Autodesk Fusion 360 part; units mm, degrees
(part 7 of 18)
  line L4400 (196.1354, -58.294) -> (195.8306, -58.294)
  line L4401 (195.8306, -58.8002) -> (196.1354, -58.8002)
  line L4402 (195.8306, -56.7954) -> (196.1354, -56.7954)
  line L4403 (196.1354, -56.7954) -> (196.1354, -57.3016)
  line L4404 (195.8306, -57.3016) -> (195.8306, -56.7954)
  line L4405 (196.1354, -57.3016) -> (195.8306, -57.3016)
  line L4406 (198.9116, -20.2852) -> (198.9116, -20.6114)
  line L4407 (198.9116, -18.7589) -> (198.9116, -19.0849)
  line L4408 (196.0592, -18.7589) -> (198.9116, -18.7589)
  line L4409 (196.0592, -20.6114) -> (198.9116, -20.6114)
  line L4410 (196.514, -20.6112) -> (196.514, -18.7588)
  line L4411 (196.1354, -20.6874) -> (196.1354, -20.1812)
  line L4412 (196.1354, -20.1812) -> (195.8306, -20.1812)
  line L4413 (195.8306, -20.1812) -> (195.8306, -20.6874)
  line L4414 (195.8306, -20.6874) -> (196.1354, -20.6874)
  line L4415 (195.8306, -19.1888) -> (195.8306, -18.6826)
  line L4416 (195.8306, -18.6826) -> (196.1354, -18.6826)
  line L4417 (196.1354, -19.1888) -> (195.8306, -19.1888)
  line L4418 (196.1354, -18.6826) -> (196.1354, -19.1888)
  line L4419 (202.7186, -3.1004) -> (203.5186, -3.1004)
  line L4420 (202.1581, -3.1) -> (201.3582, -3.1)
  line L4421 (202.7186, -4.5201) -> (203.5186, -4.5201)
  line L4422 (202.1581, -4.5196) -> (201.3582, -4.5196)
  line L4423 (203.8283, -3.4103) -> (203.8283, -4.2103)
  line L4424 (201.0484, -4.2098) -> (201.0484, -3.4098)
  arc A623 (201.3582, -4.5196) -> (201.0484, -4.2098) centre (201.3583, -4.2097) cw
  arc A624 (201.0484, -3.4098) -> (201.3582, -3.1) centre (201.3583, -3.4099) cw
  arc A625 (203.5185, -3.1004) -> (203.8283, -3.4103) centre (203.5184, -3.4104) cw
  arc A626 (203.8283, -4.2102) -> (203.5185, -4.5201) centre (203.5184, -4.2102) cw
  line L4425 (200.8136, -6.0214) -> (201.6136, -6.0214)
  line L4426 (200.2531, -6.021) -> (199.4532, -6.021)
  line L4427 (200.8136, -7.4411) -> (201.6136, -7.4411)
  line L4428 (200.2531, -7.4406) -> (199.4532, -7.4406)
  line L4429 (201.9233, -6.3313) -> (201.9233, -7.1313)
  line L4430 (199.1434, -7.1308) -> (199.1434, -6.3308)
  arc A627 (199.4532, -7.4406) -> (199.1434, -7.1308) centre (199.4533, -7.1307) cw
  arc A628 (199.1434, -6.3308) -> (199.4532, -6.021) centre (199.4533, -6.3309) cw
  arc A629 (201.6135, -6.0214) -> (201.9233, -6.3313) centre (201.6134, -6.3314) cw
  arc A630 (201.9233, -7.1312) -> (201.6135, -7.4411) centre (201.6134, -7.1312) cw
  line L4431 (205.4602, -5.5356) -> (204.6602, -5.5356)
  line L4432 (206.0207, -5.536) -> (206.8207, -5.536)
  line L4433 (205.4602, -4.1159) -> (204.6602, -4.1159)
  line L4434 (206.0207, -4.1164) -> (206.8207, -4.1164)
  line L4435 (204.3505, -5.2258) -> (204.3505, -4.4257)
  line L4436 (207.1304, -4.4262) -> (207.1304, -5.2263)
  arc A631 (206.8206, -4.1164) -> (207.1304, -4.4262) centre (206.8205, -4.4263) cw
  arc A632 (207.1304, -5.2262) -> (206.8206, -5.536) centre (206.8205, -5.2261) cw
  arc A633 (204.6603, -5.5356) -> (204.3505, -5.2258) centre (204.6604, -5.2257) cw
  arc A634 (204.3505, -4.4258) -> (204.6603, -4.1159) centre (204.6605, -4.4259) cw
  line L4437 (-3.8371, -11.3611) -> (-0.0088, -11.3611)
  line L4438 (-0.009, 0.4389) -> (-3.8371, 0.439)
  line L4439 (8.163, 0.4389) -> (8.163, -11.3611)
  line L4440 (-3.837, -11.3611) -> (-3.8371, -8.5269)
  line L4441 (1.1469, -8.2551) -> (1.1469, -2.6671)
  line L4442 (-3.8371, -11.3611) -> (-0.0088, -11.3611)
  line L4443 (4.3347, -11.3611) -> (8.163, -11.3611)
  line L4444 (8.163, 0.4389) -> (4.3348, 0.4389)
  line L4445 (0.1309, -0.6731) -> (0.1309, -1.4861)
  line L4446 (4.1949, -0.6731) -> (4.1949, -1.4861)
  line L4447 (4.3347, -11.3611) -> (8.163, -11.3611)
  line L4448 (0.1309, -9.5124) -> (0.1309, -10.2489)
  line L4449 (4.1949, -10.2489) -> (4.1949, -9.2711)
  line L4450 (-3.8371, -7.4753) -> (-3.8371, -3.4469)
  line L4451 (-3.8371, -2.3953) -> (-3.8371, 0.4389)
  arc A635 (1.1469, -3.6831) -> (1.1469, -7.2391) centre (2.1413, -5.4611) cw
  line L4452 (195.842, -3.345) -> (195.842, -5.545)
  line L4453 (195.8344, -5.588) -> (196.8504, -5.588)
  line L4454 (196.8504, -5.588) -> (196.8504, -3.302)
  line L4455 (196.8504, -3.302) -> (195.8344, -3.302)
  arc A636 (195.3213, -3.1737) -> (195.0724, -3.1725) centre (195.1968, -3.1737) ccw
  arc A637 (195.0724, -3.175) -> (195.3213, -3.1737) centre (195.1968, -3.1737) ccw
  line L4456 (177.1674, -3.048) -> (172.3373, -3.048)
  line L4457 (177.1674, -5.588) -> (177.1674, -3.048)
  line L4458 (177.1674, -5.588) -> (172.3373, -5.588)
  line L4459 (172.3373, -5.588) -> (172.3373, -3.048)
  line L4460 (181.2044, -1.3566) -> (181.2044, -3.0235)
  line L4461 (181.2044, 2.4608) -> (181.2044, 0.9765)
  line L4462 (190.1444, -1.3566) -> (190.1444, -3.0235)
  line L4463 (190.1444, 2.411) -> (190.1444, 0.9765)
  line L4464 (181.2044, 2.4608) -> (190.1444, 2.411)
  line L4465 (200.2342, -1.2444) -> (199.2753, -1.2444)
  line L4466 (199.2753, -1.2444) -> (199.2753, -2.5656)
  line L4467 (199.2753, -2.5656) -> (200.2342, -2.5656)
  line L4468 (201.0866, -1.2444) -> (202.0455, -1.2444)
  line L4469 (202.0455, -1.2444) -> (202.0455, -2.5656)
  line L4470 (202.0455, -2.5656) -> (201.0866, -2.5656)
  line L4471 (213.977, -5.1867) -> (214.6507, -5.1867)
  line L4472 (214.6507, -5.1867) -> (214.6507, -5.8604)
  line L4473 (213.977, -12.3392) -> (214.6507, -12.3392)
  line L4474 (214.6507, -12.3392) -> (214.6507, -11.6655)
  line L4475 (208.172, -5.1867) -> (207.4983, -5.1867)
  line L4476 (207.4983, -5.1867) -> (207.4983, -5.8604)
  line L4477 (208.172, -12.3392) -> (207.4983, -12.3392)
  line L4478 (207.4983, -12.3392) -> (207.4983, -11.6655)
  arc A638 (207.1096, -6.1629) -> (206.9597, -6.1629) centre (207.0347, -6.1629) ccw
  arc A639 (206.9597, -6.1629) -> (207.1096, -6.1629) centre (207.0347, -6.1629) ccw
  line L4479 (188.1326, -7.3916) -> (189.0915, -7.3916)
  line L4480 (189.0915, -7.3916) -> (189.0915, -6.0704)
  line L4481 (189.0915, -6.0704) -> (188.1326, -6.0704)
  line L4482 (187.2802, -7.3916) -> (186.3213, -7.3916)
  line L4483 (186.3213, -7.3916) -> (186.3213, -6.0704)
  line L4484 (186.3213, -6.0704) -> (187.2802, -6.0704)
  line L4485 (182.7082, -6.0704) -> (181.7493, -6.0704)
  line L4486 (181.7493, -6.0704) -> (181.7493, -7.3916)
  line L4487 (181.7493, -7.3916) -> (182.7082, -7.3916)
  line L4488 (183.5606, -6.0704) -> (184.5195, -6.0704)
  line L4489 (184.5195, -6.0704) -> (184.5195, -7.3916)
  line L4490 (184.5195, -7.3916) -> (183.5606, -7.3916)
  line L4491 (208.6489, -3.8645) -> (208.6489, -0.7644)
  line L4492 (211.749, -0.7644) -> (208.6489, -0.7644)
  line L4493 (211.7477, -3.8645) -> (211.7477, -0.7644)
  line L4494 (208.6489, -3.8886) -> (209.4871, -3.8886)
  line L4495 (210.9095, -3.8886) -> (211.7477, -3.8886)
  arc A640 (209.5125, -3.8886) -> (210.9095, -3.8886) centre (210.211, -4.1061) cw
  arc A641 (212.2667, -3.8099) -> (212.0665, -3.8099) centre (212.1666, -3.8099) ccw
  arc A642 (212.0665, -3.8099) -> (212.2667, -3.8099) centre (212.1666, -3.8099) ccw
  line L4496 (141.7615, -77.4607) -> (141.7615, -77.7869)
  line L4497 (141.7615, -75.9344) -> (141.7615, -76.2604)
  line L4498 (138.9091, -75.9344) -> (141.7615, -75.9344)
  line L4499 (138.9091, -77.7869) -> (141.7615, -77.7869)
  line L4500 (139.3639, -77.7867) -> (139.3639, -75.9343)
  line L4501 (138.9853, -77.863) -> (138.9853, -77.3568)
  line L4502 (138.6805, -77.3568) -> (138.6805, -77.863)
  line L4503 (138.9853, -77.3568) -> (138.6805, -77.3568)
  line L4504 (138.6805, -77.863) -> (138.9853, -77.863)
  line L4505 (138.6805, -76.3644) -> (138.6805, -75.8582)
  line L4506 (138.9853, -75.8582) -> (138.9853, -76.3644)
  line L4507 (138.6805, -75.8582) -> (138.9853, -75.8582)
  line L4508 (138.9853, -76.3644) -> (138.6805, -76.3644)
  line L4509 (141.7615, -20.2852) -> (141.7615, -20.6114)
  line L4510 (141.7615, -18.7589) -> (141.7615, -19.0849)
  line L4511 (138.9091, -18.7589) -> (141.7615, -18.7589)
  line L4512 (138.9091, -20.6114) -> (141.7615, -20.6114)
  line L4513 (139.3639, -20.6112) -> (139.3639, -18.7588)
  line L4514 (138.6805, -20.6874) -> (138.9853, -20.6874)
  line L4515 (138.9853, -20.1812) -> (138.6805, -20.1812)
  line L4516 (138.6805, -20.1812) -> (138.6805, -20.6874)
  line L4517 (138.9853, -20.6874) -> (138.9853, -20.1812)
  line L4518 (138.6805, -19.1888) -> (138.6805, -18.6826)
  line L4519 (138.9853, -18.6826) -> (138.9853, -19.1888)
  line L4520 (138.6805, -18.6826) -> (138.9853, -18.6826)
  line L4521 (138.9853, -19.1888) -> (138.6805, -19.1888)
  line L4522 (141.7615, -39.3352) -> (141.7615, -39.6614)
  line L4523 (141.7615, -37.8089) -> (141.7615, -38.135)
  line L4524 (138.9091, -37.8089) -> (141.7615, -37.8089)
  line L4525 (138.9091, -39.6614) -> (141.7615, -39.6614)
  line L4526 (139.3639, -39.6613) -> (139.3639, -37.8089)
  line L4527 (138.6805, -39.2313) -> (138.6805, -39.7375)
  line L4528 (138.9853, -39.7375) -> (138.9853, -39.2313)
  line L4529 (138.6805, -39.7375) -> (138.9853, -39.7375)
  line L4530 (138.9853, -39.2313) -> (138.6805, -39.2313)
  line L4531 (138.6805, -38.2389) -> (138.6805, -37.7327)
  line L4532 (138.9853, -38.2389) -> (138.6805, -38.2389)
  line L4533 (138.9853, -37.7327) -> (138.9853, -38.2389)
  line L4534 (138.6805, -37.7327) -> (138.9853, -37.7327)
  line L4535 (141.7615, -58.3979) -> (141.7615, -58.7242)
  line L4536 (141.7615, -56.8716) -> (141.7615, -57.1977)
  line L4537 (138.9091, -56.8716) -> (141.7615, -56.8716)
  line L4538 (138.9091, -58.7242) -> (141.7615, -58.7242)
  line L4539 (139.3639, -58.724) -> (139.3639, -56.8716)
  line L4540 (138.9853, -58.294) -> (138.6805, -58.294)
  line L4541 (138.6805, -58.8002) -> (138.9853, -58.8002)
  line L4542 (138.9853, -58.8002) -> (138.9853, -58.294)
  line L4543 (138.6805, -58.294) -> (138.6805, -58.8002)
  line L4544 (138.9853, -57.3016) -> (138.6805, -57.3016)
  line L4545 (138.9853, -56.7954) -> (138.9853, -57.3016)
  line L4546 (138.6805, -57.3016) -> (138.6805, -56.7954)
  line L4547 (138.6805, -56.7954) -> (138.9853, -56.7954)
  line L4548 (160.8115, -20.2852) -> (160.8115, -20.6114)
  line L4549 (160.8115, -18.7589) -> (160.8115, -19.0849)
  line L4550 (157.9591, -18.7589) -> (160.8115, -18.7589)
  line L4551 (157.9591, -20.6114) -> (160.8115, -20.6114)
  line L4552 (158.4139, -20.6112) -> (158.4139, -18.7588)
  line L4553 (157.7305, -20.6874) -> (158.0353, -20.6874)
  line L4554 (158.0353, -20.1812) -> (157.7305, -20.1812)
  line L4555 (157.7305, -20.1812) -> (157.7305, -20.6874)
  line L4556 (158.0353, -20.6874) -> (158.0353, -20.1812)
  line L4557 (158.0353, -18.6826) -> (158.0353, -19.1888)
  line L4558 (157.7305, -18.6826) -> (158.0353, -18.6826)
  line L4559 (157.7305, -19.1888) -> (157.7305, -18.6826)
  line L4560 (158.0353, -19.1888) -> (157.7305, -19.1888)
  line L4561 (160.8115, -77.4607) -> (160.8115, -77.7869)
  line L4562 (160.8115, -75.9344) -> (160.8115, -76.2604)
  line L4563 (157.9591, -75.9344) -> (160.8115, -75.9344)
  line L4564 (157.9591, -77.7869) -> (160.8115, -77.7869)
  line L4565 (158.4139, -77.7867) -> (158.4139, -75.9343)
  line L4566 (158.0353, -77.863) -> (158.0353, -77.3568)
  line L4567 (157.7305, -77.863) -> (158.0353, -77.863)
  line L4568 (158.0353, -77.3568) -> (157.7305, -77.3568)
  line L4569 (157.7305, -77.3568) -> (157.7305, -77.863)
  line L4570 (157.7305, -76.3644) -> (157.7305, -75.8582)
  line L4571 (158.0353, -76.3644) -> (157.7305, -76.3644)
  line L4572 (157.7305, -75.8582) -> (158.0353, -75.8582)
  line L4573 (158.0353, -75.8582) -> (158.0353, -76.3644)
  line L4574 (160.8115, -58.3979) -> (160.8115, -58.7242)
  line L4575 (160.8115, -56.8716) -> (160.8115, -57.1977)
  line L4576 (157.9591, -56.8716) -> (160.8115, -56.8716)
  line L4577 (157.9591, -58.7242) -> (160.8115, -58.7242)
  line L4578 (158.4139, -58.724) -> (158.4139, -56.8716)
  line L4579 (158.0353, -58.8002) -> (158.0353, -58.294)
  line L4580 (158.0353, -58.294) -> (157.7305, -58.294)
  line L4581 (157.7305, -58.8002) -> (158.0353, -58.8002)
  line L4582 (157.7305, -58.294) -> (157.7305, -58.8002)
  line L4583 (157.7305, -56.7954) -> (158.0353, -56.7954)
  line L4584 (157.7305, -57.3016) -> (157.7305, -56.7954)
  line L4585 (158.0353, -57.3016) -> (157.7305, -57.3016)
  line L4586 (158.0353, -56.7954) -> (158.0353, -57.3016)
  line L4587 (160.8115, -39.3352) -> (160.8115, -39.6614)
  line L4588 (160.8115, -37.8089) -> (160.8115, -38.135)
  line L4589 (157.9591, -37.8089) -> (160.8115, -37.8089)
  line L4590 (157.9591, -39.6614) -> (160.8115, -39.6614)
  line L4591 (158.4139, -39.6613) -> (158.4139, -37.8089)
  line L4592 (158.0353, -39.7375) -> (158.0353, -39.2313)
  line L4593 (157.7305, -39.2313) -> (157.7305, -39.7375)
  line L4594 (157.7305, -39.7375) -> (158.0353, -39.7375)
  line L4595 (158.0353, -39.2313) -> (157.7305, -39.2313)
  line L4596 (158.0353, -37.7327) -> (158.0353, -38.2389)
  line L4597 (158.0353, -38.2389) -> (157.7305, -38.2389)
  line L4598 (157.7305, -37.7327) -> (158.0353, -37.7327)
  line L4599 (157.7305, -38.2389) -> (157.7305, -37.7327)
  line L4600 (179.8616, -20.2852) -> (179.8616, -20.6114)
  line L4601 (179.8616, -18.7589) -> (179.8616, -19.0849)
  line L4602 (177.0092, -18.7589) -> (179.8616, -18.7589)
  line L4603 (177.0091, -20.6114) -> (179.8616, -20.6114)
  line L4604 (177.464, -20.6112) -> (177.464, -18.7588)
  line L4605 (176.7806, -20.6874) -> (177.0854, -20.6874)
  line L4606 (177.0854, -20.6874) -> (177.0854, -20.1812)
  line L4607 (177.0854, -20.1812) -> (176.7806, -20.1812)
  line L4608 (176.7806, -20.1812) -> (176.7806, -20.6874)
  line L4609 (177.0854, -19.1888) -> (176.7806, -19.1888)
  line L4610 (176.7806, -18.6826) -> (177.0854, -18.6826)
  line L4611 (176.7806, -19.1888) -> (176.7806, -18.6826)
  line L4612 (177.0854, -18.6826) -> (177.0854, -19.1888)
  line L4613 (179.8616, -77.4607) -> (179.8616, -77.7869)
  line L4614 (179.8616, -75.9344) -> (179.8616, -76.2604)
  line L4615 (177.0092, -75.9344) -> (179.8616, -75.9344)
  line L4616 (177.0091, -77.7869) -> (179.8616, -77.7869)
  line L4617 (177.464, -77.7867) -> (177.464, -75.9343)
  line L4618 (177.0854, -77.863) -> (177.0854, -77.3568)
  line L4619 (176.7806, -77.3568) -> (176.7806, -77.863)
  line L4620 (176.7806, -77.863) -> (177.0854, -77.863)
  line L4621 (177.0854, -77.3568) -> (176.7806, -77.3568)
  line L4622 (176.7806, -75.8582) -> (177.0854, -75.8582)
  line L4623 (177.0854, -75.8582) -> (177.0854, -76.3644)
  line L4624 (176.7806, -76.3644) -> (176.7806, -75.8582)
  line L4625 (177.0854, -76.3644) -> (176.7806, -76.3644)
  line L4626 (179.8616, -58.3979) -> (179.8616, -58.7242)
  line L4627 (179.8616, -56.8716) -> (179.8616, -57.1977)
  line L4628 (177.0092, -56.8716) -> (179.8616, -56.8716)
  line L4629 (177.0091, -58.7242) -> (179.8616, -58.7242)
  line L4630 (177.464, -58.724) -> (177.464, -56.8716)
  line L4631 (177.0854, -58.294) -> (176.7806, -58.294)
  line L4632 (176.7806, -58.294) -> (176.7806, -58.8002)
  line L4633 (176.7806, -58.8002) -> (177.0854, -58.8002)
  line L4634 (177.0854, -58.8002) -> (177.0854, -58.294)
  line L4635 (176.7806, -56.7954) -> (177.0854, -56.7954)
  line L4636 (177.0854, -57.3016) -> (176.7806, -57.3016)
  line L4637 (177.0854, -56.7954) -> (177.0854, -57.3016)
  line L4638 (176.7806, -57.3016) -> (176.7806, -56.7954)
  line L4639 (179.8616, -39.3352) -> (179.8616, -39.6614)
  line L4640 (179.8616, -37.8089) -> (179.8616, -38.135)
  line L4641 (177.0092, -37.8089) -> (179.8616, -37.8089)
  line L4642 (177.0091, -39.6614) -> (179.8616, -39.6614)
  line L4643 (177.464, -39.6613) -> (177.464, -37.8089)
  line L4644 (176.7806, -39.7375) -> (177.0854, -39.7375)
  line L4645 (177.0854, -39.2313) -> (176.7806, -39.2313)
  line L4646 (176.7806, -39.2313) -> (176.7806, -39.7375)
  line L4647 (177.0854, -39.7375) -> (177.0854, -39.2313)
  line L4648 (176.7806, -38.2389) -> (176.7806, -37.7327)
  line L4649 (177.0854, -38.2389) -> (176.7806, -38.2389)
  line L4650 (177.0854, -37.7327) -> (177.0854, -38.2389)
  line L4651 (176.7806, -37.7327) -> (177.0854, -37.7327)
  line L4652 (103.6614, -77.4607) -> (103.6614, -77.7869)
  line L4653 (103.6614, -75.9344) -> (103.6614, -76.2604)
  line L4654 (100.809, -75.9344) -> (103.6614, -75.9344)
  line L4655 (100.809, -77.7869) -> (103.6614, -77.7869)
  line L4656 (101.2638, -77.7867) -> (101.2638, -75.9343)
  line L4657 (100.8852, -77.863) -> (100.8852, -77.3568)
  line L4658 (100.5804, -77.3568) -> (100.5804, -77.863)
  line L4659 (100.5804, -77.863) -> (100.8852, -77.863)
  line L4660 (100.8852, -77.3568) -> (100.5804, -77.3568)
  line L4661 (100.5804, -75.8582) -> (100.8852, -75.8582)
  line L4662 (100.5804, -76.3644) -> (100.5804, -75.8582)
  line L4663 (100.8852, -75.8582) -> (100.8852, -76.3644)
  line L4664 (100.8852, -76.3644) -> (100.5804, -76.3644)
  line L4665 (103.6614, -58.3979) -> (103.6614, -58.7242)
  line L4666 (103.6614, -56.8716) -> (103.6614, -57.1977)
  line L4667 (100.809, -56.8716) -> (103.6614, -56.8716)
  line L4668 (100.809, -58.7242) -> (103.6614, -58.7242)
  line L4669 (101.2638, -58.724) -> (101.2638, -56.8716)
  line L4670 (100.8852, -58.294) -> (100.5804, -58.294)
  line L4671 (100.5804, -58.8002) -> (100.8852, -58.8002)
  line L4672 (100.5804, -58.294) -> (100.5804, -58.8002)
  line L4673 (100.8852, -58.8002) -> (100.8852, -58.294)
  line L4674 (100.8852, -56.7954) -> (100.8852, -57.3016)
  line L4675 (100.5804, -56.7954) -> (100.8852, -56.7954)
  line L4676 (100.5804, -57.3016) -> (100.5804, -56.7954)
  line L4677 (100.8852, -57.3016) -> (100.5804, -57.3016)
  line L4678 (103.6614, -20.2852) -> (103.6614, -20.6114)
  line L4679 (103.6614, -18.7589) -> (103.6614, -19.0849)
  line L4680 (100.809, -18.7589) -> (103.6614, -18.7589)
  line L4681 (100.809, -20.6114) -> (103.6614, -20.6114)
  line L4682 (101.2638, -20.6112) -> (101.2638, -18.7588)
  line L4683 (100.5804, -20.1812) -> (100.5804, -20.6874)
  line L4684 (100.8852, -20.1812) -> (100.5804, -20.1812)
  line L4685 (100.5804, -20.6874) -> (100.8852, -20.6874)
  line L4686 (100.8852, -20.6874) -> (100.8852, -20.1812)
  line L4687 (100.8852, -19.1888) -> (100.5804, -19.1888)
  line L4688 (100.5804, -19.1888) -> (100.5804, -18.6826)
  line L4689 (100.8852, -18.6826) -> (100.8852, -19.1888)
  line L4690 (100.5804, -18.6826) -> (100.8852, -18.6826)
  line L4691 (103.6614, -39.3352) -> (103.6614, -39.6614)
  line L4692 (103.6614, -37.8089) -> (103.6614, -38.135)
  line L4693 (100.809, -37.8089) -> (103.6614, -37.8089)
  line L4694 (100.809, -39.6614) -> (103.6614, -39.6614)
  line L4695 (101.2638, -39.6613) -> (101.2638, -37.8089)
  line L4696 (100.5804, -39.2313) -> (100.5804, -39.7375)
  line L4697 (100.8852, -39.7375) -> (100.8852, -39.2313)
  line L4698 (100.8852, -39.2313) -> (100.5804, -39.2313)
  line L4699 (100.5804, -39.7375) -> (100.8852, -39.7375)
  line L4700 (100.8852, -37.7327) -> (100.8852, -38.2389)
  line L4701 (100.5804, -38.2389) -> (100.5804, -37.7327)
  line L4702 (100.8852, -38.2389) -> (100.5804, -38.2389)
  line L4703 (100.5804, -37.7327) -> (100.8852, -37.7327)
  line L4704 (122.7115, -20.2852) -> (122.7115, -20.6114)
  line L4705 (122.7115, -18.7589) -> (122.7115, -19.0849)
  line L4706 (119.8591, -18.7589) -> (122.7115, -18.7589)
  line L4707 (119.859, -20.6114) -> (122.7115, -20.6114)
  line L4708 (120.3138, -20.6112) -> (120.3138, -18.7588)
  line L4709 (119.6304, -20.6874) -> (119.9352, -20.6874)
  line L4710 (119.6304, -20.1812) -> (119.6304, -20.6874)
  line L4711 (119.9352, -20.1812) -> (119.6304, -20.1812)
  line L4712 (119.9352, -20.6874) -> (119.9352, -20.1812)
  line L4713 (119.6304, -19.1888) -> (119.6304, -18.6826)
  line L4714 (119.9352, -18.6826) -> (119.9352, -19.1888)
  line L4715 (119.6304, -18.6826) -> (119.9352, -18.6826)
  line L4716 (119.9352, -19.1888) -> (119.6304, -19.1888)
  line L4717 (122.7115, -58.3979) -> (122.7115, -58.7242)
  line L4718 (122.7115, -56.8716) -> (122.7115, -57.1977)
  line L4719 (119.8591, -56.8716) -> (122.7115, -56.8716)
  line L4720 (119.859, -58.7242) -> (122.7115, -58.7242)
  line L4721 (120.3138, -58.724) -> (120.3138, -56.8716)
  line L4722 (119.6304, -58.8002) -> (119.9352, -58.8002)
  line L4723 (119.9352, -58.294) -> (119.6304, -58.294)
  line L4724 (119.9352, -58.8002) -> (119.9352, -58.294)
  line L4725 (119.6304, -58.294) -> (119.6304, -58.8002)
  line L4726 (119.9352, -57.3016) -> (119.6304, -57.3016)
  line L4727 (119.9352, -56.7954) -> (119.9352, -57.3016)
  line L4728 (119.6304, -56.7954) -> (119.9352, -56.7954)
  line L4729 (119.6304, -57.3016) -> (119.6304, -56.7954)
  line L4730 (122.7115, -39.3352) -> (122.7115, -39.6614)
  line L4731 (122.7115, -37.8089) -> (122.7115, -38.135)
  line L4732 (119.8591, -37.8089) -> (122.7115, -37.8089)
  line L4733 (119.859, -39.6614) -> (122.7115, -39.6614)
  line L4734 (120.3138, -39.6613) -> (120.3138, -37.8089)
  line L4735 (119.6304, -39.7375) -> (119.9352, -39.7375)
  line L4736 (119.6304, -39.2313) -> (119.6304, -39.7375)
  line L4737 (119.9352, -39.2313) -> (119.6304, -39.2313)
  line L4738 (119.9352, -39.7375) -> (119.9352, -39.2313)
  line L4739 (119.6304, -37.7327) -> (119.9352, -37.7327)
  line L4740 (119.9352, -38.2389) -> (119.6304, -38.2389)
  line L4741 (119.6304, -38.2389) -> (119.6304, -37.7327)
  line L4742 (119.9352, -37.7327) -> (119.9352, -38.2389)
  line L4743 (122.7115, -77.4607) -> (122.7115, -77.7869)
  line L4744 (122.7115, -75.9344) -> (122.7115, -76.2604)
  line L4745 (119.8591, -75.9344) -> (122.7115, -75.9344)
  line L4746 (119.859, -77.7869) -> (122.7115, -77.7869)
  line L4747 (120.3138, -77.7867) -> (120.3138, -75.9343)
  line L4748 (119.9352, -77.3568) -> (119.6304, -77.3568)
  line L4749 (119.9352, -77.863) -> (119.9352, -77.3568)
  line L4750 (119.6304, -77.3568) -> (119.6304, -77.863)
  line L4751 (119.6304, -77.863) -> (119.9352, -77.863)
  line L4752 (119.9352, -76.3644) -> (119.6304, -76.3644)
  line L4753 (119.9352, -75.8582) -> (119.9352, -76.3644)
  line L4754 (119.6304, -76.3644) -> (119.6304, -75.8582)
  line L4755 (119.6304, -75.8582) -> (119.9352, -75.8582)
  line L4756 (8.4112, -77.4607) -> (8.4112, -77.7869)
  line L4757 (8.4112, -75.9344) -> (8.4112, -76.2604)
  line L4758 (5.5588, -75.9344) -> (8.4112, -75.9344)
  line L4759 (5.5588, -77.7869) -> (8.4112, -77.7869)
  line L4760 (6.0136, -77.7867) -> (6.0136, -75.9343)
  line L4761 (5.635, -77.3568) -> (5.3302, -77.3568)
  line L4762 (5.3302, -77.863) -> (5.635, -77.863)
  line L4763 (5.3302, -77.3568) -> (5.3302, -77.863)
  line L4764 (5.635, -77.863) -> (5.635, -77.3568)
  line L4765 (5.3302, -76.3644) -> (5.3302, -75.8582)
  line L4766 (5.3302, -75.8582) -> (5.635, -75.8582)
  line L4767 (5.635, -76.3644) -> (5.3302, -76.3644)
  line L4768 (5.635, -75.8582) -> (5.635, -76.3644)
  line L4769 (27.4613, -77.4607) -> (27.4613, -77.7869)
  line L4770 (27.4613, -75.9344) -> (27.4613, -76.2604)
  line L4771 (24.6089, -75.9344) -> (27.4613, -75.9344)
  line L4772 (24.6088, -77.7869) -> (27.4613, -77.7869)
  line L4773 (25.0637, -77.7867) -> (25.0637, -75.9343)
  line L4774 (24.3803, -77.3568) -> (24.3803, -77.863)
  line L4775 (24.6851, -77.3568) -> (24.3803, -77.3568)
  line L4776 (24.3803, -77.863) -> (24.6851, -77.863)
  line L4777 (24.6851, -77.863) -> (24.6851, -77.3568)
  line L4778 (24.6851, -75.8582) -> (24.6851, -76.3644)
  line L4779 (24.3803, -76.3644) -> (24.3803, -75.8582)
  line L4780 (24.3803, -75.8582) -> (24.6851, -75.8582)
  line L4781 (24.6851, -76.3644) -> (24.3803, -76.3644)
  line L4782 (46.5113, -77.4607) -> (46.5113, -77.7869)
  line L4783 (46.5113, -75.9344) -> (46.5113, -76.2604)
  line L4784 (43.6589, -75.9344) -> (46.5113, -75.9344)
  line L4785 (43.6589, -77.7869) -> (46.5113, -77.7869)
  line L4786 (44.1137, -77.7867) -> (44.1137, -75.9343)
  line L4787 (43.4303, -77.3568) -> (43.4303, -77.863)
  line L4788 (43.4303, -77.863) -> (43.7351, -77.863)
  line L4789 (43.7351, -77.863) -> (43.7351, -77.3568)
  line L4790 (43.7351, -77.3568) -> (43.4303, -77.3568)
  line L4791 (43.7351, -75.8582) -> (43.7351, -76.3644)
  line L4792 (43.4303, -75.8582) -> (43.7351, -75.8582)
  line L4793 (43.4303, -76.3644) -> (43.4303, -75.8582)
  line L4794 (43.7351, -76.3644) -> (43.4303, -76.3644)
  line L4795 (65.5613, -20.2852) -> (65.5613, -20.6114)
  line L4796 (65.5613, -18.7589) -> (65.5613, -19.0849)
  line L4797 (62.7089, -18.7589) -> (65.5613, -18.7589)
  line L4798 (62.7089, -20.6114) -> (65.5613, -20.6114)
  line L4799 (63.1637, -20.6112) -> (63.1637, -18.7588)
  line L4800 (62.7851, -20.6874) -> (62.7851, -20.1812)
  line L4801 (62.4803, -20.1812) -> (62.4803, -20.6874)
  line L4802 (62.4803, -20.6874) -> (62.7851, -20.6874)
  line L4803 (62.7851, -20.1812) -> (62.4803, -20.1812)
  line L4804 (62.4803, -18.6826) -> (62.7851, -18.6826)
  line L4805 (62.4803, -19.1888) -> (62.4803, -18.6826)
  line L4806 (62.7851, -18.6826) -> (62.7851, -19.1888)
  line L4807 (62.7851, -19.1888) -> (62.4803, -19.1888)
  line L4808 (65.5613, -77.4607) -> (65.5613, -77.7869)
  line L4809 (65.5613, -75.9344) -> (65.5613, -76.2604)
  line L4810 (62.7089, -75.9344) -> (65.5613, -75.9344)
  line L4811 (62.7089, -77.7869) -> (65.5613, -77.7869)
  line L4812 (63.1637, -77.7867) -> (63.1637, -75.9343)
  line L4813 (62.7851, -77.3568) -> (62.4803, -77.3568)
  line L4814 (62.4803, -77.863) -> (62.7851, -77.863)
  line L4815 (62.4803, -77.3568) -> (62.4803, -77.863)
  line L4816 (62.7851, -77.863) -> (62.7851, -77.3568)
  line L4817 (62.7851, -76.3644) -> (62.4803, -76.3644)
  line L4818 (62.4803, -75.8582) -> (62.7851, -75.8582)
  line L4819 (62.7851, -75.8582) -> (62.7851, -76.3644)
  line L4820 (62.4803, -76.3644) -> (62.4803, -75.8582)
  line L4821 (65.5613, -39.3352) -> (65.5613, -39.6614)
  line L4822 (65.5613, -37.8089) -> (65.5613, -38.135)
  line L4823 (62.7089, -37.8089) -> (65.5613, -37.8089)
  line L4824 (62.7089, -39.6614) -> (65.5613, -39.6614)
  line L4825 (63.1637, -39.6613) -> (63.1637, -37.8089)
  line L4826 (62.7851, -39.7375) -> (62.7851, -39.2313)
  line L4827 (62.4803, -39.7375) -> (62.7851, -39.7375)
  line L4828 (62.7851, -39.2313) -> (62.4803, -39.2313)
  line L4829 (62.4803, -39.2313) -> (62.4803, -39.7375)
  line L4830 (62.4803, -38.2389) -> (62.4803, -37.7327)
  line L4831 (62.7851, -38.2389) -> (62.4803, -38.2389)
  line L4832 (62.7851, -37.7327) -> (62.7851, -38.2389)
  line L4833 (62.4803, -37.7327) -> (62.7851, -37.7327)
  line L4834 (65.5613, -58.3979) -> (65.5613, -58.7242)
  line L4835 (65.5613, -56.8716) -> (65.5613, -57.1977)
  line L4836 (62.7089, -56.8716) -> (65.5613, -56.8716)
  line L4837 (62.7089, -58.7242) -> (65.5613, -58.7242)
  line L4838 (63.1637, -58.724) -> (63.1637, -56.8716)
  line L4839 (62.7851, -58.294) -> (62.4803, -58.294)
  line L4840 (62.4803, -58.8002) -> (62.7851, -58.8002)
  line L4841 (62.7851, -58.8002) -> (62.7851, -58.294)
  line L4842 (62.4803, -58.294) -> (62.4803, -58.8002)
  line L4843 (62.7851, -56.7954) -> (62.7851, -57.3016)
  line L4844 (62.7851, -57.3016) -> (62.4803, -57.3016)
  line L4845 (62.4803, -56.7954) -> (62.7851, -56.7954)
  line L4846 (62.4803, -57.3016) -> (62.4803, -56.7954)
  line L4847 (84.6114, -39.3352) -> (84.6114, -39.6614)
  line L4848 (84.6114, -37.8089) -> (84.6114, -38.135)
  line L4849 (81.759, -37.8089) -> (84.6114, -37.8089)
  line L4850 (81.759, -39.6614) -> (84.6114, -39.6614)
  line L4851 (82.2138, -39.6613) -> (82.2138, -37.8089)
  line L4852 (81.5304, -39.2313) -> (81.5304, -39.7375)
  line L4853 (81.5304, -39.7375) -> (81.8352, -39.7375)
  line L4854 (81.8352, -39.2313) -> (81.5304, -39.2313)
  line L4855 (81.8352, -39.7375) -> (81.8352, -39.2313)
  line L4856 (81.5304, -37.7327) -> (81.8352, -37.7327)
  line L4857 (81.8352, -38.2389) -> (81.5304, -38.2389)
  line L4858 (81.5304, -38.2389) -> (81.5304, -37.7327)
  line L4859 (81.8352, -37.7327) -> (81.8352, -38.2389)
  line L4860 (84.6114, -77.4607) -> (84.6114, -77.7869)
  line L4861 (84.6114, -75.9344) -> (84.6114, -76.2604)
  line L4862 (81.759, -75.9344) -> (84.6114, -75.9344)
  line L4863 (81.759, -77.7869) -> (84.6114, -77.7869)
  line L4864 (82.2138, -77.7867) -> (82.2138, -75.9343)
  line L4865 (81.8352, -77.863) -> (81.8352, -77.3568)
  line L4866 (81.5304, -77.3568) -> (81.5304, -77.863)
  line L4867 (81.5304, -77.863) -> (81.8352, -77.863)
  line L4868 (81.8352, -77.3568) -> (81.5304, -77.3568)
  line L4869 (81.8352, -75.8582) -> (81.8352, -76.3644)
  line L4870 (81.5304, -75.8582) -> (81.8352, -75.8582)
  line L4871 (81.8352, -76.3644) -> (81.5304, -76.3644)
  line L4872 (81.5304, -76.3644) -> (81.5304, -75.8582)
  line L4873 (84.6114, -20.2852) -> (84.6114, -20.6114)
  line L4874 (84.6114, -18.7589) -> (84.6114, -19.0849)
  line L4875 (81.759, -18.7589) -> (84.6114, -18.7589)
  line L4876 (81.759, -20.6114) -> (84.6114, -20.6114)
  line L4877 (82.2138, -20.6112) -> (82.2138, -18.7588)
  line L4878 (81.5304, -20.1812) -> (81.5304, -20.6874)
  line L4879 (81.8352, -20.6874) -> (81.8352, -20.1812)
  line L4880 (81.5304, -20.6874) -> (81.8352, -20.6874)
  line L4881 (81.8352, -20.1812) -> (81.5304, -20.1812)
  line L4882 (81.5304, -18.6826) -> (81.8352, -18.6826)
  line L4883 (81.5304, -19.1888) -> (81.5304, -18.6826)
  line L4884 (81.8352, -18.6826) -> (81.8352, -19.1888)
  line L4885 (81.8352, -19.1888) -> (81.5304, -19.1888)
  line L4886 (84.6114, -58.3979) -> (84.6114, -58.7242)
  line L4887 (84.6114, -56.8716) -> (84.6114, -57.1977)
  line L4888 (81.759, -56.8716) -> (84.6114, -56.8716)
  line L4889 (81.759, -58.7242) -> (84.6114, -58.7242)
  line L4890 (82.2138, -58.724) -> (82.2138, -56.8716)
  line L4891 (81.5304, -58.294) -> (81.5304, -58.8002)
  line L4892 (81.5304, -58.8002) -> (81.8352, -58.8002)
  line L4893 (81.8352, -58.8002) -> (81.8352, -58.294)
  line L4894 (81.8352, -58.294) -> (81.5304, -58.294)
  line L4895 (81.8352, -57.3016) -> (81.5304, -57.3016)
  line L4896 (81.5304, -57.3016) -> (81.5304, -56.7954)
  line L4897 (81.8352, -56.7954) -> (81.8352, -57.3016)
  line L4898 (81.5304, -56.7954) -> (81.8352, -56.7954)
  line L4899 (8.4112, -58.3979) -> (8.4112, -58.7242)
  line L4900 (8.4112, -56.8716) -> (8.4112, -57.1977)
  line L4901 (5.5588, -56.8716) -> (8.4112, -56.8716)
  line L4902 (5.5588, -58.7242) -> (8.4112, -58.7242)
  line L4903 (6.0136, -58.724) -> (6.0136, -56.8716)
  line L4904 (5.3302, -58.8002) -> (5.635, -58.8002)
  line L4905 (5.635, -58.8002) -> (5.635, -58.294)
  line L4906 (5.635, -58.294) -> (5.3302, -58.294)
  line L4907 (5.3302, -58.294) -> (5.3302, -58.8002)
  line L4908 (5.635, -57.3016) -> (5.3302, -57.3016)
  line L4909 (5.3302, -56.7954) -> (5.635, -56.7954)
  line L4910 (5.635, -56.7954) -> (5.635, -57.3016)
  line L4911 (5.3302, -57.3016) -> (5.3302, -56.7954)
  line L4912 (8.4112, -20.2852) -> (8.4112, -20.6114)
  line L4913 (8.4112, -18.7589) -> (8.4112, -19.0849)
  line L4914 (5.5588, -18.7589) -> (8.4112, -18.7589)
  line L4915 (5.5588, -20.6114) -> (8.4112, -20.6114)
  line L4916 (6.0136, -20.6112) -> (6.0136, -18.7588)
  line L4917 (5.3302, -20.6874) -> (5.635, -20.6874)
  line L4918 (5.635, -20.1812) -> (5.3302, -20.1812)
  line L4919 (5.3302, -20.1812) -> (5.3302, -20.6874)
  line L4920 (5.635, -20.6874) -> (5.635, -20.1812)
  line L4921 (5.3302, -19.1888) -> (5.3302, -18.6826)
  line L4922 (5.3302, -18.6826) -> (5.635, -18.6826)
  line L4923 (5.635, -19.1888) -> (5.3302, -19.1888)
  line L4924 (5.635, -18.6826) -> (5.635, -19.1888)
  line L4925 (8.4112, -39.3352) -> (8.4112, -39.6614)
  line L4926 (8.4112, -37.8089) -> (8.4112, -38.135)
  line L4927 (5.5588, -37.8089) -> (8.4112, -37.8089)
  line L4928 (5.5588, -39.6614) -> (8.4112, -39.6614)
  line L4929 (6.0136, -39.6613) -> (6.0136, -37.8089)
  line L4930 (5.635, -39.7375) -> (5.635, -39.2313)
  line L4931 (5.3302, -39.7375) -> (5.635, -39.7375)
  line L4932 (5.635, -39.2313) -> (5.3302, -39.2313)
  line L4933 (5.3302, -39.2313) -> (5.3302, -39.7375)
  line L4934 (5.635, -37.7327) -> (5.635, -38.2389)
  line L4935 (5.635, -38.2389) -> (5.3302, -38.2389)
  line L4936 (5.3302, -38.2389) -> (5.3302, -37.7327)
  line L4937 (5.3302, -37.7327) -> (5.635, -37.7327)
  line L4938 (27.4613, -39.3352) -> (27.4613, -39.6614)
  line L4939 (27.4613, -37.8089) -> (27.4613, -38.135)
  line L4940 (24.6089, -37.8089) -> (27.4613, -37.8089)
  line L4941 (24.6088, -39.6614) -> (27.4613, -39.6614)
  line L4942 (25.0637, -39.6613) -> (25.0637, -37.8089)
  line L4943 (24.6851, -39.2313) -> (24.3803, -39.2313)
  line L4944 (24.3803, -39.7375) -> (24.6851, -39.7375)
  line L4945 (24.3803, -39.2313) -> (24.3803, -39.7375)
  line L4946 (24.6851, -39.7375) -> (24.6851, -39.2313)
  line L4947 (24.3803, -38.2389) -> (24.3803, -37.7327)
  line L4948 (24.3803, -37.7327) -> (24.6851, -37.7327)
  line L4949 (24.6851, -38.2389) -> (24.3803, -38.2389)
  line L4950 (24.6851, -37.7327) -> (24.6851, -38.2389)
  line L4951 (27.4613, -20.2852) -> (27.4613, -20.6114)
  line L4952 (27.4613, -18.7589) -> (27.4613, -19.0849)
  line L4953 (24.6089, -18.7589) -> (27.4613, -18.7589)
  line L4954 (24.6088, -20.6114) -> (27.4613, -20.6114)
  line L4955 (25.0637, -20.6112) -> (25.0637, -18.7588)
  line L4956 (24.3803, -20.6874) -> (24.6851, -20.6874)
  line L4957 (24.6851, -20.6874) -> (24.6851, -20.1812)
  line L4958 (24.3803, -20.1812) -> (24.3803, -20.6874)
  line L4959 (24.6851, -20.1812) -> (24.3803, -20.1812)
  line L4960 (24.3803, -19.1888) -> (24.3803, -18.6826)
  line L4961 (24.6851, -19.1888) -> (24.3803, -19.1888)
  line L4962 (24.3803, -18.6826) -> (24.6851, -18.6826)
  line L4963 (24.6851, -18.6826) -> (24.6851, -19.1888)
  line L4964 (27.4613, -58.3979) -> (27.4613, -58.7242)
  line L4965 (27.4613, -56.8716) -> (27.4613, -57.1977)
  line L4966 (24.6089, -56.8716) -> (27.4613, -56.8716)
  line L4967 (24.6088, -58.7242) -> (27.4613, -58.7242)
  line L4968 (25.0637, -58.724) -> (25.0637, -56.8716)
  line L4969 (24.6851, -58.294) -> (24.3803, -58.294)
  line L4970 (24.6851, -58.8002) -> (24.6851, -58.294)
  line L4971 (24.3803, -58.294) -> (24.3803, -58.8002)
  line L4972 (24.3803, -58.8002) -> (24.6851, -58.8002)
  line L4973 (24.3803, -56.7954) -> (24.6851, -56.7954)
  line L4974 (24.3803, -57.3016) -> (24.3803, -56.7954)
  line L4975 (24.6851, -57.3016) -> (24.3803, -57.3016)
  line L4976 (24.6851, -56.7954) -> (24.6851, -57.3016)
  line L4977 (46.5113, -20.2852) -> (46.5113, -20.6114)
  line L4978 (46.5113, -18.7589) -> (46.5113, -19.0849)
  line L4979 (43.6589, -18.7589) -> (46.5113, -18.7589)
  line L4980 (43.6589, -20.6114) -> (46.5113, -20.6114)
  line L4981 (44.1137, -20.6112) -> (44.1137, -18.7588)
  line L4982 (43.4303, -20.1812) -> (43.4303, -20.6874)
  line L4983 (43.4303, -20.6874) -> (43.7351, -20.6874)
  line L4984 (43.7351, -20.1812) -> (43.4303, -20.1812)
  line L4985 (43.7351, -20.6874) -> (43.7351, -20.1812)
  line L4986 (43.7351, -18.6826) -> (43.7351, -19.1888)
  line L4987 (43.7351, -19.1888) -> (43.4303, -19.1888)
  line L4988 (43.4303, -18.6826) -> (43.7351, -18.6826)
  line L4989 (43.4303, -19.1888) -> (43.4303, -18.6826)
  line L4990 (46.5113, -58.3979) -> (46.5113, -58.7242)
  line L4991 (46.5113, -56.8716) -> (46.5113, -57.1977)
  line L4992 (43.6589, -56.8716) -> (46.5113, -56.8716)
  line L4993 (43.6589, -58.7242) -> (46.5113, -58.7242)
  line L4994 (44.1137, -58.724) -> (44.1137, -56.8716)
  line L4995 (43.7351, -58.8002) -> (43.7351, -58.294)
  line L4996 (43.7351, -58.294) -> (43.4303, -58.294)
  line L4997 (43.4303, -58.294) -> (43.4303, -58.8002)
  line L4998 (43.4303, -58.8002) -> (43.7351, -58.8002)
  line L4999 (43.7351, -56.7954) -> (43.7351, -57.3016)
  line L5000 (43.4303, -57.3016) -> (43.4303, -56.7954)
  line L5001 (43.7351, -57.3016) -> (43.4303, -57.3016)
  line L5002 (43.4303, -56.7954) -> (43.7351, -56.7954)
  line L5003 (46.5113, -39.3352) -> (46.5113, -39.6614)
  line L5004 (46.5113, -37.8089) -> (46.5113, -38.135)
  line L5005 (43.6589, -37.8089) -> (46.5113, -37.8089)
  line L5006 (43.6589, -39.6614) -> (46.5113, -39.6614)
  line L5007 (44.1137, -39.6613) -> (44.1137, -37.8089)
  line L5008 (43.4303, -39.7375) -> (43.7351, -39.7375)
  line L5009 (43.7351, -39.7375) -> (43.7351, -39.2313)
  line L5010 (43.4303, -39.2313) -> (43.4303, -39.7375)
  line L5011 (43.7351, -39.2313) -> (43.4303, -39.2313)
  line L5012 (43.7351, -38.2389) -> (43.4303, -38.2389)
  line L5013 (43.7351, -37.7327) -> (43.7351, -38.2389)
  line L5014 (43.4303, -38.2389) -> (43.4303, -37.7327)
  line L5015 (43.4303, -37.7327) -> (43.7351, -37.7327)
  line L5016 (217.9616, -20.2852) -> (217.9616, -20.6114)
  line L5017 (217.9616, -18.7589) -> (217.9616, -19.0849)
  line L5018 (215.1092, -18.7589) -> (217.9616, -18.7589)
  line L5019 (215.1092, -20.6114) -> (217.9616, -20.6114)
  line L5020 (215.564, -20.6112) -> (215.564, -18.7588)
  line L5021 (214.8806, -20.1812) -> (214.8806, -20.6874)
  line L5022 (215.1854, -20.6874) -> (215.1854, -20.1812)
  line L5023 (214.8806, -20.6874) -> (215.1854, -20.6874)
  line L5024 (215.1854, -20.1812) -> (214.8806, -20.1812)
  line L5025 (215.1854, -19.1888) -> (214.8806, -19.1888)
  line L5026 (214.8806, -19.1888) -> (214.8806, -18.6826)
  line L5027 (215.1854, -18.6826) -> (215.1854, -19.1888)
  line L5028 (214.8806, -18.6826) -> (215.1854, -18.6826)
  line L5029 (217.9616, -77.4607) -> (217.9616, -77.7869)
  line L5030 (217.9616, -75.9344) -> (217.9616, -76.2604)
  line L5031 (215.1092, -75.9344) -> (217.9616, -75.9344)
  line L5032 (215.1092, -77.7869) -> (217.9616, -77.7869)
  line L5033 (215.564, -77.7867) -> (215.564, -75.9343)
  line L5034 (215.1854, -77.3568) -> (214.8806, -77.3568)
  line L5035 (215.1854, -77.863) -> (215.1854, -77.3568)
  line L5036 (214.8806, -77.863) -> (215.1854, -77.863)
  line L5037 (214.8806, -77.3568) -> (214.8806, -77.863)
  line L5038 (215.1854, -76.3644) -> (214.8806, -76.3644)
  line L5039 (214.8806, -75.8582) -> (215.1854, -75.8582)
  line L5040 (215.1854, -75.8582) -> (215.1854, -76.3644)
  line L5041 (214.8806, -76.3644) -> (214.8806, -75.8582)
  line L5042 (217.9616, -58.3979) -> (217.9616, -58.7242)
  line L5043 (217.9616, -56.8716) -> (217.9616, -57.1977)
  line L5044 (215.1092, -56.8716) -> (217.9616, -56.8716)
  line L5045 (215.1092, -58.7242) -> (217.9616, -58.7242)
  line L5046 (215.564, -58.724) -> (215.564, -56.8716)
  line L5047 (215.1854, -58.294) -> (214.8806, -58.294)
  line L5048 (215.1854, -58.8002) -> (215.1854, -58.294)
  line L5049 (214.8806, -58.8002) -> (215.1854, -58.8002)
  line L5050 (214.8806, -58.294) -> (214.8806, -58.8002)
  line L5051 (214.8806, -57.3016) -> (214.8806, -56.7954)
  line L5052 (215.1854, -56.7954) -> (215.1854, -57.3016)
  line L5053 (214.8806, -56.7954) -> (215.1854, -56.7954)
  line L5054 (215.1854, -57.3016) -> (214.8806, -57.3016)
  line L5055 (217.9616, -39.3352) -> (217.9616, -39.6614)
  line L5056 (217.9616, -37.8089) -> (217.9616, -38.135)
  line L5057 (215.1092, -37.8089) -> (217.9616, -37.8089)
  line L5058 (215.1092, -39.6614) -> (217.9616, -39.6614)
  line L5059 (215.564, -39.6613) -> (215.564, -37.8089)
  line L5060 (215.1854, -39.7375) -> (215.1854, -39.2313)
  line L5061 (214.8806, -39.7375) -> (215.1854, -39.7375)
  line L5062 (215.1854, -39.2313) -> (214.8806, -39.2313)
  line L5063 (214.8806, -39.2313) -> (214.8806, -39.7375)
  line L5064 (214.8806, -37.7327) -> (215.1854, -37.7327)
  line L5065 (214.8806, -38.2389) -> (214.8806, -37.7327)
  line L5066 (215.1854, -37.7327) -> (215.1854, -38.2389)
  line L5067 (215.1854, -38.2389) -> (214.8806, -38.2389)
  line L5068 (198.9116, -39.3352) -> (198.9116, -39.6614)
  line L5069 (198.9116, -37.8089) -> (198.9116, -38.135)
  line L5070 (196.0592, -37.8089) -> (198.9116, -37.8089)
  line L5071 (196.0592, -39.6614) -> (198.9116, -39.6614)
  line L5072 (196.514, -39.6613) -> (196.514, -37.8089)
  line L5073 (196.1354, -39.7375) -> (196.1354, -39.2313)
  line L5074 (195.8306, -39.7375) -> (196.1354, -39.7375)
  line L5075 (195.8306, -39.2313) -> (195.8306, -39.7375)
  line L5076 (196.1354, -39.2313) -> (195.8306, -39.2313)
  line L5077 (195.8306, -38.2389) -> (195.8306, -37.7327)
  line L5078 (196.1354, -37.7327) -> (196.1354, -38.2389)
  line L5079 (196.1354, -38.2389) -> (195.8306, -38.2389)
  line L5080 (195.8306, -37.7327) -> (196.1354, -37.7327)
  line L5081 (198.9116, -77.4607) -> (198.9116, -77.7869)
  line L5082 (198.9116, -75.9344) -> (198.9116, -76.2604)
  line L5083 (196.0592, -75.9344) -> (198.9116, -75.9344)
  line L5084 (196.0592, -77.7869) -> (198.9116, -77.7869)
  line L5085 (196.514, -77.7867) -> (196.514, -75.9343)
  line L5086 (195.8306, -77.863) -> (196.1354, -77.863)
  line L5087 (196.1354, -77.3568) -> (195.8306, -77.3568)
  line L5088 (196.1354, -77.863) -> (196.1354, -77.3568)
  line L5089 (195.8306, -77.3568) -> (195.8306, -77.863)
  line L5090 (195.8306, -75.8582) -> (196.1354, -75.8582)
  line L5091 (196.1354, -76.3644) -> (195.8306, -76.3644)
  line L5092 (195.8306, -76.3644) -> (195.8306, -75.8582)
  line L5093 (196.1354, -75.8582) -> (196.1354, -76.3644)
  line L5094 (198.9116, -58.3979) -> (198.9116, -58.7242)
  line L5095 (198.9116, -56.8716) -> (198.9116, -57.1977)
  line L5096 (196.0592, -56.8716) -> (198.9116, -56.8716)
  line L5097 (196.0592, -58.7242) -> (198.9116, -58.7242)
  line L5098 (196.514, -58.724) -> (196.514, -56.8716)
  line L5099 (196.1354, -58.8002) -> (196.1354, -58.294)
  line L5100 (195.8306, -58.294) -> (195.8306, -58.8002)
  line L5101 (196.1354, -58.294) -> (195.8306, -58.294)
  line L5102 (195.8306, -58.8002) -> (196.1354, -58.8002)
  line L5103 (196.1354, -57.3016) -> (195.8306, -57.3016)
  line L5104 (195.8306, -57.3016) -> (195.8306, -56.7954)
  line L5105 (196.1354, -56.7954) -> (196.1354, -57.3016)
  line L5106 (195.8306, -56.7954) -> (196.1354, -56.7954)
  line L5107 (198.9116, -20.2852) -> (198.9116, -20.6114)
  line L5108 (198.9116, -18.7589) -> (198.9116, -19.0849)
  line L5109 (196.0592, -18.7589) -> (198.9116, -18.7589)
  line L5110 (196.0592, -20.6114) -> (198.9116, -20.6114)
  line L5111 (196.514, -20.6112) -> (196.514, -18.7588)
  line L5112 (195.8306, -20.1812) -> (195.8306, -20.6874)
  line L5113 (196.1354, -20.6874) -> (196.1354, -20.1812)
  line L5114 (196.1354, -20.1812) -> (195.8306, -20.1812)
  line L5115 (195.8306, -20.6874) -> (196.1354, -20.6874)
  line L5116 (195.8306, -18.6826) -> (196.1354, -18.6826)
  line L5117 (196.1354, -19.1888) -> (195.8306, -19.1888)
  line L5118 (195.8306, -19.1888) -> (195.8306, -18.6826)
  line L5119 (196.1354, -18.6826) -> (196.1354, -19.1888)
  line L5120 (202.7186, -3.1004) -> (203.5186, -3.1004)
  line L5121 (202.1581, -3.1) -> (201.3582, -3.1)
  line L5122 (202.7186, -4.5201) -> (203.5186, -4.5201)
  line L5123 (202.1581, -4.5196) -> (201.3582, -4.5196)
  line L5124 (203.8283, -3.4103) -> (203.8283, -4.2103)
  line L5125 (201.0484, -4.2098) -> (201.0484, -3.4098)
  arc A643 (201.3582, -4.5196) -> (201.0484, -4.2098) centre (201.3583, -4.2097) cw
  arc A644 (201.0484, -3.4098) -> (201.3582, -3.1) centre (201.3583, -3.4099) cw
  arc A645 (203.5185, -3.1004) -> (203.8283, -3.4103) centre (203.5184, -3.4104) cw
  arc A646 (203.8283, -4.2102) -> (203.5185, -4.5201) centre (203.5184, -4.2102) cw
  line L5126 (200.8136, -6.0214) -> (201.6136, -6.0214)
  line L5127 (200.2531, -6.021) -> (199.4532, -6.021)
  line L5128 (200.8136, -7.4411) -> (201.6136, -7.4411)
  line L5129 (200.2531, -7.4406) -> (199.4532, -7.4406)
  line L5130 (201.9233, -6.3313) -> (201.9233, -7.1313)
  line L5131 (199.1434, -7.1308) -> (199.1434, -6.3308)
  arc A647 (199.4532, -7.4406) -> (199.1434, -7.1308) centre (199.4533, -7.1307) cw
  arc A648 (199.1434, -6.3308) -> (199.4532, -6.021) centre (199.4533, -6.3309) cw
  arc A649 (201.6135, -6.0214) -> (201.9233, -6.3313) centre (201.6134, -6.3314) cw
  arc A650 (201.9233, -7.1312) -> (201.6135, -7.4411) centre (201.6134, -7.1312) cw
  line L5132 (205.4602, -5.5356) -> (204.6602, -5.5356)
  line L5133 (206.0207, -5.536) -> (206.8207, -5.536)
  line L5134 (205.4602, -4.1159) -> (204.6602, -4.1159)
  line L5135 (206.0207, -4.1164) -> (206.8207, -4.1164)
  line L5136 (204.3505, -5.2258) -> (204.3505, -4.4257)
  line L5137 (207.1304, -4.4262) -> (207.1304, -5.2263)
  arc A651 (206.8206, -4.1164) -> (207.1304, -4.4262) centre (206.8205, -4.4263) cw
  arc A652 (207.1304, -5.2262) -> (206.8206, -5.536) centre (206.8205, -5.2261) cw
  arc A653 (204.6603, -5.5356) -> (204.3505, -5.2258) centre (204.6604, -5.2257) cw
  arc A654 (204.3505, -4.4258) -> (204.6603, -4.1159) centre (204.6605, -4.4259) cw
  line L5138 (-3.8371, -11.3611) -> (-0.0088, -11.3611)
  line L5139 (-0.009, 0.4389) -> (-3.8371, 0.439)
  line L5140 (8.163, 0.4389) -> (8.163, -11.3611)
  line L5141 (-3.837, -11.3611) -> (-3.8371, -8.5269)
  line L5142 (1.1469, -8.2551) -> (1.1469, -2.6671)
  line L5143 (-3.8371, -11.3611) -> (-0.0088, -11.3611)
  line L5144 (4.3347, -11.3611) -> (8.163, -11.3611)
  line L5145 (8.163, 0.4389) -> (4.3348, 0.4389)
  line L5146 (0.1309, -0.6731) -> (0.1309, -1.4861)
  line L5147 (4.1949, -0.6731) -> (4.1949, -1.4861)
  line L5148 (4.3347, -11.3611) -> (8.163, -11.3611)
  line L5149 (0.1309, -9.5124) -> (0.1309, -10.2489)
  line L5150 (4.1949, -10.2489) -> (4.1949, -9.2711)
  line L5151 (-3.8371, -7.4753) -> (-3.8371, -3.4469)
  line L5152 (-3.8371, -2.3953) -> (-3.8371, 0.4389)
  arc A655 (1.1469, -3.6831) -> (1.1469, -7.2391) centre (2.1413, -5.4611) cw
  arc A656 (-2.1624, -5.4611) -> (6.4883, -5.4611) centre (2.1629, -5.4611) ccw
  arc A657 (6.4883, -5.4611) -> (-2.1624, -5.4611) centre (2.1629, -5.4611) ccw
  arc A658 (5.5157, -5.4611) -> (-1.1899, -5.4611) centre (2.1629, -5.4611) ccw
  arc A659 (-1.1899, -5.4611) -> (5.5157, -5.4611) centre (2.1629, -5.4611) ccw
  arc A660 (5.2109, -5.4611) -> (-0.8851, -5.4611) centre (2.1629, -5.4611) ccw
  arc A661 (-0.8851, -5.4611) -> (5.2109, -5.4611) centre (2.1629, -5.4611) ccw
  line L5153 (195.842, -3.345) -> (195.842, -5.545)
  line L5154 (195.8344, -5.588) -> (196.8504, -5.588)
  line L5155 (196.8504, -5.588) -> (196.8504, -3.302)
  line L5156 (196.8504, -3.302) -> (195.8344, -3.302)
  arc A662 (195.0724, -3.175) -> (195.3213, -3.1737) centre (195.1968, -3.1737) ccw
  arc A663 (195.3213, -3.1737) -> (195.0724, -3.1725) centre (195.1968, -3.1737) ccw
  line L5157 (184.8974, -50.5184) -> (198.8974, -50.5184)
  line L5158 (198.8974, -50.5184) -> (198.8974, -64.5184)
  line L5159 (198.8974, -64.5184) -> (184.8974, -64.5184)
  line L5160 (184.8974, -64.5184) -> (184.8974, -50.5184)
  line L5161 (179.8474, -83.5812) -> (165.8473, -83.5812)
  line L5162 (165.8473, -69.5811) -> (179.8474, -69.5811)
  line L5163 (179.8474, -69.5811) -> (179.8474, -83.5812)
  line L5164 (165.8473, -83.5812) -> (165.8473, -69.5811)
  line L5165 (179.8474, -64.5184) -> (165.8473, -64.5184)
  line L5166 (179.8474, -50.5184) -> (179.8474, -64.5184)
  line L5167 (165.8473, -50.5184) -> (179.8474, -50.5184)
  line L5168 (165.8473, -64.5184) -> (165.8473, -50.5184)
  line L5169 (165.8473, -31.4557) -> (179.8474, -31.4557)
  line L5170 (179.8474, -45.4557) -> (165.8473, -45.4557)
  line L5171 (165.8473, -45.4557) -> (165.8473, -31.4557)
  line L5172 (179.8474, -31.4557) -> (179.8474, -45.4557)
  line L5173 (165.8473, -26.4057) -> (165.8473, -12.4056)
  line L5174 (165.8473, -12.4056) -> (179.8474, -12.4056)
  line L5175 (179.8474, -12.4056) -> (179.8474, -26.4057)
  line L5176 (179.8474, -26.4057) -> (165.8473, -26.4057)
  line L5177 (160.7973, -69.5811) -> (160.7973, -83.5812)
  line L5178 (160.7973, -83.5812) -> (146.7973, -83.5812)
  line L5179 (146.7973, -83.5812) -> (146.7973, -69.5811)
  line L5180 (146.7973, -69.5811) -> (160.7973, -69.5811)
  line L5181 (146.7973, -45.4557) -> (146.7973, -31.4557)
  line L5182 (160.7973, -31.4557) -> (160.7973, -45.4557)
  line L5183 (160.7973, -45.4557) -> (146.7973, -45.4557)
  line L5184 (146.7973, -31.4557) -> (160.7973, -31.4557)
  line L5185 (146.7973, -64.5184) -> (146.7973, -50.5184)
  line L5186 (160.7973, -64.5184) -> (146.7973, -64.5184)
  line L5187 (160.7973, -50.5184) -> (160.7973, -64.5184)
  line L5188 (146.7973, -50.5184) -> (160.7973, -50.5184)
  line L5189 (160.7973, -26.4057) -> (146.7973, -26.4057)
  line L5190 (160.7973, -12.4056) -> (160.7973, -26.4057)
  line L5191 (146.7973, -12.4056) -> (160.7973, -12.4056)
  line L5192 (146.7973, -26.4057) -> (146.7973, -12.4056)
  line L5193 (127.7473, -64.5184) -> (127.7473, -50.5184)
  line L5194 (127.7473, -50.5184) -> (141.7473, -50.5184)
  line L5195 (141.7473, -50.5184) -> (141.7473, -64.5184)
  line L5196 (141.7473, -64.5184) -> (127.7473, -64.5184)
  line L5197 (127.7473, -31.4557) -> (141.7473, -31.4557)
  line L5198 (127.7473, -45.4557) -> (127.7473, -31.4557)
  line L5199 (141.7473, -31.4557) -> (141.7473, -45.4557)
  line L5200 (141.7473, -45.4557) -> (127.7473, -45.4557)
  line L5201 (141.7473, -12.4056) -> (141.7473, -26.4057)
  line L5202 (141.7473, -26.4057) -> (127.7473, -26.4057)
  line L5203 (127.7473, -12.4056) -> (141.7473, -12.4056)
  line L5204 (127.7473, -26.4057) -> (127.7473, -12.4056)
  line L5205 (127.7473, -69.5811) -> (141.7473, -69.5811)
  line L5206 (141.7473, -83.5812) -> (127.7473, -83.5812)
  line L5207 (127.7473, -83.5812) -> (127.7473, -69.5811)
  line L5208 (141.7473, -69.5811) -> (141.7473, -83.5812)
  line L5209 (122.6972, -83.5812) -> (108.6972, -83.5812)
  line L5210 (122.6972, -69.5811) -> (122.6972, -83.5812)
  line L5211 (108.6972, -83.5812) -> (108.6972, -69.5811)
  line L5212 (108.6972, -69.5811) -> (122.6972, -69.5811)
  line L5213 (122.6972, -50.5184) -> (122.6972, -64.5184)
  line L5214 (108.6972, -64.5184) -> (108.6972, -50.5184)
  line L5215 (122.6972, -64.5184) -> (108.6972, -64.5184)
  line L5216 (108.6972, -50.5184) -> (122.6972, -50.5184)
  line L5217 (122.6972, -12.4056) -> (122.6972, -26.4057)
  line L5218 (108.6972, -12.4056) -> (122.6972, -12.4056)
  line L5219 (122.6972, -26.4057) -> (108.6972, -26.4057)
  line L5220 (108.6972, -26.4057) -> (108.6972, -12.4056)
  line L5221 (122.6972, -31.4557) -> (122.6972, -45.4557)